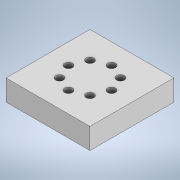
# Autodesk Inventor part: Part13
Saved by Autodesk Inventor 2020 (Build 240168000, 168)
## iProperties
Created: 2019-12-31
Part Number: Part13
Material: Generic
Document SubType Name: Modeling
Designer: tdmp4
Density: 1 g/cm^3
Appearance: Default
Author: tdmp4
Autodesk Inventor part; units mm, degrees
ref_plane "YZ Plane" through (0, 0, 0) normal (1, 0, 0) x (0, 1, 0)
ref_plane "XZ Plane" through (0, 0, 0) normal (0, 1, 0) x (-1, 0, 0)
ref_plane "XY Plane" through (0, 0, 0) normal (0, 0, 1) x (1, 0, 0)
sketch "Sketch1" plane through (0, 0, 0) normal (0, 1, 0) x (-1, 0, 0)
  line L0 (0, 0) -> (38.1, 0)
  line L1 (38.1, 0) -> (38.1, -38.1)
  line L2 (38.1, -38.1) -> (0, -38.1)
  line L3 (0, -38.1) -> (0, 0)
  circle A0 centre (28.829, -19.05) radius 1.7859
  circle A1 centre (9.271, -19.05) radius 1.7859
  circle A2 centre (19.05, -28.829) radius 1.7859
  circle A3 centre (19.05, -9.271) radius 1.7859
  circle A4 centre (12.1352, -12.1352) radius 1.7859
  circle A5 centre (12.1352, -25.9648) radius 1.7859
  circle A6 centre (25.9648, -25.9648) radius 1.7859
  circle A7 centre (25.9648, -12.1352) radius 1.7859
  dimension "d0" = 38.1
  dimension "d1" = 38.1
  dimension "d3" = 3.5719
  dimension "d4" = 3.5719
  dimension "d5" = 3.5719
  dimension "d6" = 3.5719
  dimension "d8" = 3.5719
  dimension "d9" = 3.5719
  dimension "d10" = 3.5719
  dimension "d11" = 3.5719
  constraints: 8 centre point, 8 end point, 2 parallel, 1 horizontal, 1 perpendicular
  measures "d0" distance of L1.end L2.end
  measures "d1" distance of L2.end L0.start
  measures "d3" diameter of A0
  measures "d4" diameter of A1
  measures "d5" diameter of A2
  measures "d6" diameter of A3
  measures "d8" diameter of A4
  measures "d9" diameter of A5
  measures "d10" diameter of A6
  measures "d11" diameter of A7
extrude "Extrusion1" add sketch "Sketch1" along normal blind 9.525
body "Solid1"
